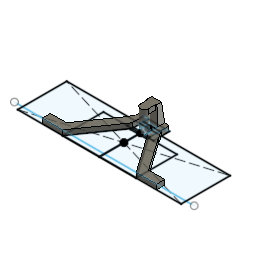
GlassMaskAntiFg-v1 (Autodesk Fusion 360 design; units mm, degrees)
Autodesk Fusion 360 part; units mm, degrees
sketch "スケッチ1" plane through (0, 0, 0) normal (0, 1, 0) x (1, 0, 0)
  line L0 (50, -15) -> (-50, -15)
  line L1 (-50, -15) -> (-50, 15)
  line L2 (-50, 15) -> (50, 15)
  line L3 (50, 15) -> (50, -15)
  line L4 (50, -15) -> (-50, 15) construction
  line L5 (-50, -15) -> (50, 15) construction
  line L6 (0, -15) -> (22.5, -15)
  line L7 (22.5, -15) -> (22.5, 10)
  line L8 (22.5, 10) -> (0, 10)
  line L9 (0, 10) -> (0, -15)
  line L10 (0, 10) -> (-22.5, 10)
  line L11 (-22.5, 10) -> (-22.5, -15)
  line L12 (-22.5, -15) -> (0, -15)
  line L13 (0, -15) -> (0, 10)
  line L14 (5, 9) -> (-5, 9)
  line L15 (-5, 9) -> (-5, 11)
  line L16 (-5, 11) -> (5, 11)
  line L17 (5, 11) -> (5, 9)
  line L18 (5, 9) -> (-5, 11) construction
  line L19 (-5, 9) -> (5, 11) construction
  line L20 (-5, 10) -> (-22.5, -15)
  line L21 (5, 10) -> (22.5, -15)
  line L22 (-55, -12) -> (55, -12)
  line L23 (5, 14) -> (-5, 14)
  line L24 (-5, 14) -> (-5, 16)
  line L25 (-5, 16) -> (5, 16)
  line L26 (5, 16) -> (5, 14)
  line L27 (5, 14) -> (-5, 16) construction
  line L28 (-5, 14) -> (5, 16) construction
  circle A0 centre (0, 12.5) radius 2.5
  line L29 (-5, 15) -> (5, 15)
  line L30 (5, 15) -> (5, 17)
  line L31 (5, 17) -> (-5, 17)
  line L32 (-5, 17) -> (-5, 15)
  line L33 (-5, 17) -> (5, 17)
  line L34 (5, 17) -> (5, 20)
  line L35 (5, 20) -> (-5, 20)
  line L36 (-5, 20) -> (-5, 17)
  line L37 (-5, 10) -> (-8, 10)
  line L38 (-8, 10) -> (-8, 20)
  line L39 (-8, 20) -> (-5, 20)
  line L40 (-5, 20) -> (-5, 10)
  line L41 (5, 10) -> (8, 10)
  line L42 (8, 10) -> (8, 20)
  line L43 (8, 20) -> (5, 20)
  line L44 (5, 20) -> (5, 10)
  line L45 (-2.5, 18) -> (2.5, 18)
  line L46 (2.5, 18) -> (2.5, 12.5)
  line L47 (2.5, 12.5) -> (-2.5, 12.5)
  line L48 (-2.5, 12.5) -> (-2.5, 18)
  point P0 (0, 10)
  point P1 (0, 15)
  dimension "d1" = 100
  dimension "d2" = 30
  dimension "d3" = 25
  dimension "d4" = 22.5
  dimension "d5" = 25
  dimension "d6" = 22.5
  dimension "d7" = 2
  dimension "d8" = 10
  dimension "d61" = 5
  dimension "d62" = 10
  dimension "d63" = 2
  dimension "d64" = 10
  dimension "d65" = 3
  dimension "d66" = 3
  dimension "d67" = 3
  dimension "d83" = 5
  dimension "d84" = 5.5
  constraint perpendicular L0 L1
  constraint parallel L0 L2
  constraint parallel L1 L3
  constraint horizontal L0
  constraint coincident L4 origin
  constraint coincident L5 origin
  constraint horizontal L6
  constraint vertical L7
  constraint horizontal L8
  constraint vertical L9
  constraint midpoint L0 L6.start
  constraint horizontal L10
  constraint vertical L11
  constraint horizontal L12
  constraint vertical L13
  constraint perpendicular L14 L15
  constraint parallel L14 L16
  constraint parallel L15 L17
  constraint horizontal L14
  constraint coincident L18 P0
  constraint coincident L19 P0
  constraint coincident P0 L8.end
  constraint midpoint L15 L20.start
  constraint midpoint L17 L21.start
  constraint perpendicular L3 L22
  constraint perpendicular L23 L24
  constraint parallel L23 L25
  constraint parallel L24 L26
  constraint horizontal L23
  constraint coincident L27 P1
  constraint coincident L28 P1
  constraint midpoint L2 P1
  constraint midpoint L24 L29.start
  constraint horizontal L29
  constraint vertical L30
  constraint horizontal L31
  constraint vertical L32
  constraint horizontal L33
  constraint vertical L34
  constraint horizontal L35
  constraint vertical L36
  constraint horizontal L37
  constraint vertical L38
  constraint horizontal L39
  constraint vertical L40
  constraint horizontal L41
  constraint vertical L42
  constraint horizontal L43
  constraint vertical L44
  constraint horizontal L45
  constraint vertical L46
  constraint horizontal L47
  constraint vertical L48
  measures "d1" distance of L1.end L2.end
  measures "d2" distance of L0.end L1.end
  measures "d3" distance of L6.start P0
  measures "d4" distance of L6.start L6.end L0.start
  measures "d5" distance of P0 L6.start
  measures "d6" distance of P0 L10.end
  measures "d7" distance of L14.end L15.end
  measures "d8" distance of L15.end L16.end
  measures "d61" diameter of A0
  measures "d62" distance of L29.start L29.end
  measures "d63" distance of L29.start L31.end
  measures "d64" distance of L31.end L30.end
  measures "d65" distance of L31.end L35.end
  measures "d66" distance of L20.start L37.end
  measures "d67" distance of L21.start L41.end
  measures "d83" distance of L45.start L45.end
  measures "d84" distance of L45.start L47.end
extrude "押し出し14" add sketch "スケッチ1" along normal blind 3 contours L0 L3 L7 L22 | L7 L21 L22 | L2 L3 L7 L8 L22 L42 | L7 L8 L21 L22 L41 | L0 L1 L11 L22 | L11 L20 L22 | L2 L8 L17 L26 L41 L42 L44 | L2 L26 L30 L34 L42 L43 L44 | L1 L2 L10 L11 L22 L38 | L10 L11 L20 L22 L37 | L2 L10 L15 L24 L37 L38 L40 | L2 L24 L32 L36 L38 L39 L40 makes body 1 at (-26.8333, 0, -5) makes body 2 at (26.8333, 0, -5)
extrude "押し出し15" add sketch "スケッチ1" along normal blind 13 contours L16 A0 | L16 A0 L47 | L31 L33 L34 L35 L36 L40 L44 L45 L46 L48 | L23 A0 L47 | L23 A0 | L31 L33 L45 L46 L48 bodies 1 2 makes body 3 at (2.4876, 4.3333, -12.2511)
sketch "スケッチ14" plane through (0, 0, -17) normal (0, 0, 1) x (1, 0, 0)
  line L0 (-5, 0) -> (5, 0)
  line L1 (5, 0) -> (5, 3)
  line L2 (5, 3) -> (5, 13)
  line L3 (5, 13) -> (-5, 13)
  line L4 (-5, 13) -> (-5, 3)
  line L5 (-5, 3) -> (-5, 0)
  line L6 (0, 13) -> (2.5, 13)
  line L7 (2.5, 13) -> (2.5, 10)
  line L8 (2.5, 10) -> (0, 10)
  line L9 (0, 10) -> (0, 13)
  line L10 (0, 13) -> (-2.5, 13)
  line L11 (-2.5, 13) -> (-2.5, 10)
  line L12 (-2.5, 10) -> (0, 10)
  line L13 (0, 10) -> (0, 13)
  dimension "d72" = 2.5
  dimension "d73" = 3
  dimension "d74" = 3
  constraint horizontal L6
  constraint vertical L7
  constraint horizontal L8
  constraint vertical L9
  constraint midpoint L3 L6.start
  constraint horizontal L10
  constraint vertical L11
  constraint horizontal L12
  constraint vertical L13
  measures "d72" distance of L6.start L6.end
  measures "d73" distance of L6.start L8.end
  measures "d74" distance of L6.start L8.end
extrude "押し出し16" add sketch "スケッチ14" along normal blind 4.5 contours L3 L9 L10 L11 L12 L13 | L3 L6 L7 L8 L9 L13 bodies 3 1
sketch "スケッチ15" plane through (0, 3, 0) normal (0, 1, 0) x (-1, 0, 0)
  line L0 (5, -20) -> (8, -20)
  line L1 (8, -20) -> (8, -15)
  line L2 (8, -15) -> (50, -15)
  line L3 (50, -15) -> (50, 15)
  line L4 (50, 15) -> (22.5, 15)
  line L5 (22.5, 15) -> (5, -10)
  line L6 (5, -10) -> (5, -17)
  line L7 (5, -17) -> (5, -20)
  line L8 (11.1033, -10) -> (45, -10)
  line L9 (45, -10) -> (45, 10)
  line L10 (45, 10) -> (25.1033, 10)
  line L11 (25.1033, 10) -> (11.1033, -10)
  line L12 (11.1033, -10) -> (8, -15)
  line L13 (45, 10) -> (50, 10)
  dimension "d77" = -5
  constraint coincident L1.end L2.start
  constraint coincident L3 L13.end
  constraint perpendicular L3 L13
extrude "押し出し17" cut sketch "スケッチ15" against normal blind 3 contours L2 L3 L8 L9 L12 L13 | L8 L9 L10 L11 bodies 3
sketch "スケッチ16" plane through (0, 3, 0) normal (0, 1, 0) x (-1, 0, 0)
  line L0 (-8, -15) -> (-8, -20)
  line L1 (-8, -20) -> (-5, -20)
  line L2 (-5, -20) -> (-5, -17)
  line L3 (-5, -17) -> (-5, -10)
  line L4 (-5, -10) -> (-22.5, 15)
  line L5 (-22.5, 15) -> (-50, 15)
  line L6 (-50, 15) -> (-50, -15)
  line L7 (-50, -15) -> (-8, -15)
  line L8 (-45, 10) -> (-45, -10)
  line L9 (-45, -10) -> (-11.1033, -10)
  line L10 (-11.1033, -10) -> (-25.1033, 10)
  line L11 (-25.1033, 10) -> (-45, 10)
  line L12 (-11.1033, -10) -> (-8, -15)
  line L13 (-45, 10) -> (-50, 10)
  dimension "d80" = -5
  constraint coincident L0.start L7.end
  constraint coincident L6 L13.end
  constraint perpendicular L6 L13
extrude "押し出し18" cut sketch "スケッチ16" against normal blind 3 contours L6 L7 L8 L9 L12 L13 | L8 L9 L10 L11 bodies 3
extrude "押し出し19" add sketch "スケッチ1" along normal blind 0.3 contours L2 L23 A0 L29 L46 | L2 L25 L29 L46 L48 | L23 A0 L48 | L23 A0 L47 | L23 A0 L46 | L2 L23 A0 L29 L48 | L23 A0 | L25 L31 L33 L46 L48 bodies 3
extrude "押し出し20" cut 1 faces at (50, 1, 11.6667) along direction (-1, 0, 0) blind 15 on bodies 3 bodies 3
extrude "押し出し21" cut 1 faces at (-50, 1, 13.3333) along direction (1, 0, 0) blind 15 on bodies 3 bodies 3
chamfer "面取り2" distance 2 distance2 10 1 edges at (-5, 13, -18.5) measured on face at (-0.8333, 13, -14) on bodies 3
chamfer "面取り3" distance 2 distance2 10 1 edges at (5, 13, -18.5) measured on face at (-0.8333, 13, -14) on bodies 3
chamfer "面取り4" distance 1.5 angle 45 2 edges at (-5, 1.5, -17) (5, 1.5, -17) on bodies 3
chamfer "面取り5" distance 1 angle 45 2 edges at (-8, 1.5, -20) (8, 1.5, -20) on bodies 3
equation "d4 = ( 45 / 2 ) * 1 mm"
equation "d6 = ( 45 / 2 ) * 1 mm"
